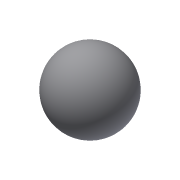
# Autodesk Inventor part: 00_bearing_ball_2mm
Saved by Autodesk Inventor 2019.4 (Build 234330000, 330)
## iProperties
Created: 2021-05-16
Part Number: 00_bearing_ball_2mm
Material: Generic
Document SubType Name: Modeling
Designer: diederichbenedict
Density: 1 g/cm^3
Appearance: Default
Author: diederichbenedict
Autodesk Inventor part; units mm, degrees
ref_plane "YZ Plane" through (0, 0, 0) normal (1, 0, 0) x (0, 1, 0)
ref_plane "XZ Plane" through (0, 0, 0) normal (0, 1, 0) x (-1, 0, 0)
ref_plane "XY Plane" through (0, 0, 0) normal (0, 0, 1) x (1, 0, 0)
sketch "Sketch1" plane through (0, 0, 0) normal (0, 1, 0) x (-1, 0, 0)
  circle A0 centre (89.4519, 43.1632) radius 1
  line L0 (90.4519, 43.1632) -> (88.4519, 43.1632)
  point P0 (0, 0)
  dimension "d0" = 2
  dimension "d0" = 2
  constraints: 2 end point, 2 point on circle, 1 centre point
  measures "d0" diameter of A0
revolve "Revolution1" add sketch "Sketch1" angle 360 about axis through (-90.4519, 0, 43.1632) along (1, 0, 0) picked at (89.7014, 43.5438) contours L0 A0
body "Solid1"
